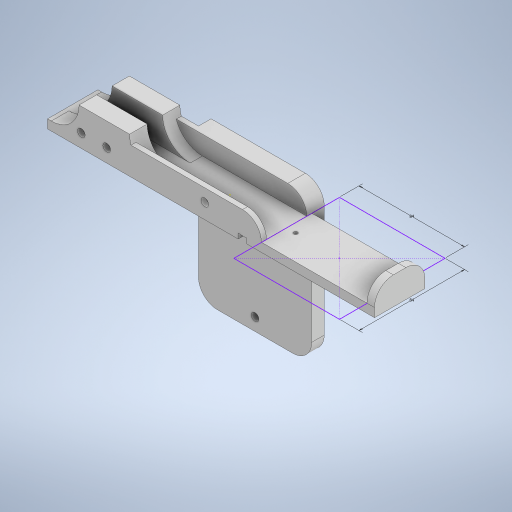
# Autodesk Inventor part: Zeitmessung_Halterung
Saved by Autodesk Inventor 2024.2 (Build 282272000, 272)
## iProperties
Created: 2023-10-20
Part Number: Zeitmessung_Halterung
Material: Generic
Document SubType Name: Modeling
Designer: Rene
Density: 1 g/cm^3
Appearance: Default
Author: Rene
Autodesk Inventor part; units mm, degrees
ref_plane "YZ Plane" through (0, 0, 0) normal (1, 0, 0) x (0, 1, 0)
ref_plane "XZ Plane" through (0, 0, 0) normal (0, 1, 0) x (-1, 0, 0)
ref_plane "XY Plane" through (0, 0, 0) normal (0, 0, 1) x (1, 0, 0)
sketch "Sketch2" plane through (0, 0, 0) normal (0, 1, 0) x (-1, 0, 0)
  line L0 (125, -20) -> (-125, -20)
  line L1 (-125, -20) -> (-125, 20)
  line L2 (-125, 20) -> (125, 20)
  line L3 (125, 20) -> (125, -20)
  line L4 (125, -20) -> (-125, 20) construction
  line L5 (-125, -20) -> (125, 20) construction
  point P0 (0, 0)
  dimension "d0" = 250
  dimension "d1" = 40
  constraints: 12 end point, 2 midpoint, 2 parallel, 1 horizontal, 1 perpendicular
  measures "d0" distance of L1.end L2.end
  measures "d1" distance of L0.end L1.end
extrude "Extrusion1" add sketch "Sketch2" along normal blind 7
sketch "Sketch5" plane through (0, 7, 0) normal (0, 1, 0) x (1, 0, 0)
  line L0 (-100, -6) -> (-59.8, -6)
  line L1 (-59.8, -6) -> (-59.8, 6.25)
  line L2 (-59.8, 6.25) -> (-100, 6.25)
  line L3 (-100, 6.25) -> (-100, -6)
  line L4 (-100, -6) -> (-59.8, 6.25) construction
  line L5 (-59.8, -6) -> (-100, 6.25) construction
  line L6 (-100, 6.5) -> (-100, -6)
  circle A0 centre (-115, 0) radius 3.5 projected
  line L7 (-125, -20) -> (125, -20) projected
  line L8 (-59.8, -6) -> (-100, -6)
  line L9 (-100, -6) -> (-100, -20)
  line L10 (-100, -20) -> (-59.8, -20)
  line L11 (-59.8, -20) -> (-59.8, -6)
  line L12 (125, 20) -> (-125, 20) projected
  line L13 (-59.8, 6.25) -> (-100, 6.25)
  line L14 (-100, 6.25) -> (-100, 20)
  line L15 (-100, 20) -> (-59.8, 20)
  line L16 (-59.8, 20) -> (-59.8, 6.25)
  point P0 (0, 0)
  point P1 (-79.9, 0.125)
  point P2 (-59.8, 20)
  point P3 (-100, 6.25)
  point P4 (-59.8, -20)
  point P5 (-111.5, 0)
  dimension "d18" = 40.2
  dimension "d19" = 12.25
  dimension "d41" = 11.5
  dimension "d42" = 40.2
  constraints: 30 end point, 6 parallel, 3 horizontal, 3 perpendicular, 3 point on line, 2 midpoint, 1 horizontal alignment, 1 other
  measures "d18" distance of L2.end L1.end
  measures "d19" distance of L1.end L0.end
  measures "d41" distance from line of point (-111.5, 0) L14
  measures "d42" distance between parallel lines of L9 L11
extrude "Extrusion4" add sketch "Sketch5" along normal blind 22 contours L0 L11 L7 L9 | L6 L14 L12 L16 L2
sketch "Sketch8" plane through (-125, 0, 20) normal (0, 0, 1) x (1, 0, 0)
  line L0 (65.2, 7) -> (25, 7) projected
  line L1 (25, 7) -> (65.2, 7)
  circle A0 centre (47.0137, 10.6993) radius 1.75
  circle A1 centre (26.8137, 10.7) radius 1.75
  line L2 (48.7637, 10.6999) -> (65.2, 10.6999)
  line L3 (65.2, 7) -> (65.2, 29) projected
  line L4 (26.8, 8.9501) -> (25, 8.9501)
  line L5 (25, 7) -> (25, 29) projected
  point P0 (125, 0)
  dimension "d30" = 3.5
  dimension "d31" = 3.5
  dimension "d32" = 16.7
  dimension "d36" = 3.7
  dimension "d44" = 1.8
  constraints: 6 end point, 3 horizontal, 2 point on line, 6 other
  measures "d36" distance from line of L0 point (26.814, 10.7)
  measures "d44" distance of L4.start L4.end
extrude "Extrusion6" cut sketch "Sketch8" against normal through all
sketch "Sketch9" plane through (0, 7, 0) normal (0, 1, 0) x (1, 0, 0)
  line L0 (61, -11.5) -> (100, -11.5)
  line L1 (100, -11.5) -> (100, 11.5)
  line L2 (100, 11.5) -> (61, 11.5)
  line L3 (61, 11.5) -> (61, -11.5)
  circle A0 centre (80.5, 0) radius 2.05 projected
  line L4 (61, -11.5) -> (100, 11.5) construction
  line L5 (100, -11.5) -> (61, 11.5) construction
  circle A1 centre (115, 0) radius 3.5 projected
  line L6 (-125, -20) -> (125, -20) projected
  line L7 (-59.8, -6) -> (-59.8, -20) projected
  line L8 (125, -20) -> (-59.8, -20)
  line L9 (-59.8, -20) -> (-59.8, -16)
  line L10 (-59.8, -16) -> (125, -16)
  line L11 (125, -16) -> (125, -20)
  line L12 (125, 20) -> (-125, 20) projected
  line L13 (125, 20) -> (-59.8, 20)
  line L14 (-59.8, 20) -> (-59.8, 16)
  line L15 (-59.8, 16) -> (125, 16)
  line L16 (125, 16) -> (125, 20)
  point P0 (0, 0)
  point P1 (-59.8, 20)
  dimension "d39" = 39
  dimension "d40" = 23
  dimension "d45" = 4
  dimension "d46" = 4
  constraints: 28 end point, 6 parallel, 3 horizontal, 3 perpendicular, 2 midpoint, 2 point on line
  measures "d39" distance of L2.end L1.end
  measures "d40" distance of L1.end L0.end
  measures "d45" distance of L8.end L9.end
  measures "d46" distance of L14.end L13.end
extrude "Extrusion7" add sketch "Sketch9" along normal blind 15 contours L7 L10 L11 L6 | L16 L15 L14 L12
fillet "Face Fillet1" radius 22 1 edges at (-100, 7, 13)
fillet "Face Fillet2" radius 21.999 1 edges at (-100, 7, -13.125)
fillet "Face Fillet3" radius 22 1 edges at (-59.8, 7, 11)
fillet "Face Fillet4" radius 21.999 1 edges at (-59.8, 7, -11.125)
sketch "Sketch10" plane through (125, 0, -20) normal (0, 0, -1) x (-1, 0, 0)
  circle A0 centre (202.9863, 10.6993) radius 1.75 projected
  line L0 (204.6029, 13.4993) -> (206.2195, 10.6993)
  line L1 (206.2195, 10.6993) -> (204.6029, 7.8993)
  line L2 (204.6029, 7.8993) -> (201.3697, 7.8993)
  line L3 (201.3697, 7.8993) -> (199.7532, 10.6993)
  line L4 (199.7532, 10.6993) -> (201.3697, 13.4993)
  line L5 (201.3697, 13.4993) -> (204.6029, 13.4993)
  circle A1 centre (223.1863, 10.7) radius 1.75 projected
  line L6 (224.8029, 13.5) -> (226.4195, 10.7)
  line L7 (226.4195, 10.7) -> (224.8029, 7.9)
  line L8 (224.8029, 7.9) -> (221.5697, 7.9)
  line L9 (221.5697, 7.9) -> (219.9532, 10.7)
  line L10 (219.9532, 10.7) -> (221.5697, 13.5)
  line L11 (221.5697, 13.5) -> (224.8029, 13.5)
  point P0 (125, 0)
  dimension "d55" = 5.6
  dimension "d56" = 5.6
  constraints: 24 end point, 2 coincident, 26 other
  measures "d55" distance between parallel lines of L2 L5
  measures "d56" distance between parallel lines of L8 L11
extrude "Extrusion8" cut sketch "Sketch10" against normal blind 5 contours A0 | L0 L1 L2 L3 L4 L5 | A1 | L6 L7 L8 L9 L10 L11
sketch "Sketch11" plane through (-125, 0, 20) normal (0, 0, 1) x (1, 0, 0)
  circle A0 centre (26.8137, 10.7) radius 1.75 projected
  circle A1 centre (26.8137, 10.7) radius 3
  circle A2 centre (47.0137, 10.6993) radius 1.75 projected
  circle A3 centre (47.0137, 10.6993) radius 3
  point P0 (125, 0)
  dimension "d59" = 6
  dimension "d60" = 6
  constraints: 2 centre point, 2 coincident
  measures "d59" diameter of A1
  measures "d60" diameter of A3
extrude "Extrusion9" cut sketch "Sketch11" against normal blind 4
sketch "Sketch24" plane through (125, 0, -20) normal (0, 0, -1) x (-1, 0, 0)
  line L0 (125, 0) -> (170, 0)
  line L1 (0, 0) -> (250, 0) projected
  line L2 (183.6567, 22) -> (0, 22) projected
  line L3 (170, 0) -> (80, 0)
  line L4 (80, 0) -> (80, 22)
  line L5 (80, 22) -> (170, 22)
  line L6 (170, 22) -> (170, 0)
  point P0 (15, 22)
  point P1 (170, 22)
  point P2 (80, 0)
  dimension "d103" = 45
  dimension "d104" = 90
  constraints: 10 end point, 2 parallel, 2 point on line, 1 horizontal, 1 perpendicular
  measures "d103" distance of L0.start L0.end
  measures "d104" distance of L4.end L5.end
extrude "Extrusion20" add sketch "Sketch24" along normal blind 10
sketch "Sketch25" plane through (0, 0, 0) normal (0, -1, 0) x (1, 0, 0)
  line L0 (-45, -30) -> (45, -30) projected
  line L1 (45, -20) -> (45, -30) projected
  line L2 (-45, -30) -> (45, -30)
  line L3 (45, -30) -> (45, -20)
  line L4 (45, -20) -> (-45, -20)
  line L5 (-45, -20) -> (-45, -30)
  point P0 (0, 0)
  constraints: 8 end point, 2 parallel, 1 horizontal, 1 perpendicular
extrude "Extrusion21" add sketch "Sketch25" along normal blind 80
sketch "Sketch28" plane through (125, 0, -30) normal (0, 0, -1) x (-1, 0, 0)
  circle A0 centre (94.9248, -27.5) radius 3.5
  line L0 (170, 22) -> (80, 22) projected
  line L1 (80, 22) -> (80, -80) projected
  point P0 (125, 0)
  point P1 (80, -29)
  dimension "d132" = 7
  dimension "d134" = 46
  dimension "d135" = 15
  constraints: 1 centre point, 1 midpoint
  measures "d132" diameter of A0
  measures "d134" distance edge to line of A0 L0
  measures "d135" distance of A0.centre point (80, -29)
extrude "Extrusion23" cut sketch "Sketch28" against normal up to surface (10 mm away)
sketch "Sketch30" plane through (0, -80, 0) normal (0, -1, 0) x (1, 0, 0)
  line L0 (45, -20) -> (45, -30) projected
  line L1 (45, -20) -> (-45, -20) projected
  line L2 (45, -30) -> (-45, -30)
  line L3 (-45, -30) -> (-45, -20)
  line L4 (-45, -20) -> (45, -20)
  line L5 (45, -20) -> (45, -30)
  point P0 (0, 0)
  constraints: 8 end point, 2 parallel, 1 horizontal, 1 perpendicular
extrude "Extrusion25" add sketch "Sketch30" along normal blind 17
sketch "Sketch31" plane through (125, 0, -30) normal (0, 0, -1) x (-1, 0, 0)
  line L0 (80, -97) -> (170, -97) projected
  line L1 (170, 22) -> (170, -97) projected
  line L2 (80, -97) -> (170, -97)
  line L3 (170, -97) -> (170, -77)
  line L4 (170, -77) -> (80, -77)
  line L5 (80, -77) -> (80, -97)
  circle A0 centre (125, -87) radius 3
  point P0 (125, 0)
  dimension "d143" = 20
  dimension "d144" = 6
  dimension "d170" = 10
  constraints: 8 end point, 2 parallel, 1 centre point, 1 horizontal, 1 perpendicular, 1 point on line
  measures "d143" distance of L3.end L2.end
  measures "d144" diameter of A0
  measures "d170" distance from line of L0 A0.centre
extrude "Extrusion26" cut sketch "Sketch31" against normal through all contours A0
sketch "Sketch35" plane through (-125, 0, 20) normal (0, 0, 1) x (1, 0, 0)
  circle A0 centre (125, 12) radius 3
  line L0 (66.3433, 22) -> (250, 22) projected
  point P0 (125, 0)
  point P1 (125.5, 22)
  point P2 (235, 22)
  dimension "d160" = 6
  dimension "d161" = 10
  constraints: 1 centre point
  measures "d160" diameter of A0
  measures "d161" distance from line of L0 A0.centre
extrude "Extrusion30" cut sketch "Sketch35" against normal blind 4
sketch "Sketch36" plane through (-45, -97, -20) normal (0, 0, 1) x (1, 0, 0)
  circle A0 centre (75.0752, 69.5) radius 3.5 projected
  line L0 (78.5752, 69.5) -> (71.5752, 69.5)
  line L1 (71.5752, 69.5) -> (71.5752, 101)
  line L2 (71.5752, 101) -> (78.5752, 101)
  line L3 (78.5752, 101) -> (78.5752, 69.5)
  point P0 (45, 97)
  point P1 (71.5752, 69.5)
  dimension "d164" = 7
  constraints: 8 end point, 2 parallel, 1 horizontal, 1 perpendicular, 2 other
  measures "d164" distance of L1.end L2.end
extrude "Extrusion31" cut sketch "Sketch36" against normal blind 4 contours A0 L1 L2 L3
sketch "Sketch37" plane through (0, 0, 0) normal (0, -1, 0) x (1, 0, 0)
  line L0 (-58.6567, 20) -> (125, 20) projected
  line L1 (26.5752, -24) -> (33.5752, -24)
  line L2 (33.5752, -24) -> (33.5752, 20)
  line L3 (33.5752, 20) -> (26.5752, 20)
  line L4 (26.5752, 20) -> (26.5752, -24)
  point P0 (0, 0)
  point P1 (0.5, 20)
  point P2 (110, 20)
  dimension "d167" = 7
  constraints: 8 end point, 2 parallel, 1 horizontal, 1 perpendicular, 1 point on line
  measures "d167" distance of L3.end L2.end
extrude "Extrusion32" cut sketch "Sketch37" against normal blind 4
fillet "Rundung5" radius 15 1 edges at (45, -97, -25)
fillet "Rundung6" radius 15 1 edges at (-45, -97, -25)
sketch "Skizze40" plane through (0, 7, 0) normal (0, 1, 0) x (1, 0, 0)
  point P0 (0, 0)
sketch "Skizze41" plane through (0, 7, 0) normal (0, 1, 0) x (1, 0, 0)
  line L0 (125, -20) -> (125, -16) projected
  line L1 (125, -20) -> (135, -20)
  line L2 (135, -20) -> (135, 20)
  line L3 (135, 20) -> (125, 20)
  line L4 (125, 20) -> (125, -20)
  point P0 (0, 0)
  dimension "d173" = 10
  constraints: 8 end point, 2 parallel, 1 horizontal, 1 perpendicular
  measures "d173" distance of L3.end L2.end
extrude "Extrusion33" add sketch "Skizze41" against normal blind 7
sketch "Skizze42" plane through (0, 7, 0) normal (0, 1, 0) x (1, 0, 0)
  line L0 (45, -42) -> (129, -42)
  line L1 (129, -42) -> (129, 42)
  line L2 (129, 42) -> (45, 42)
  line L3 (45, 42) -> (45, -42)
  line L4 (45, -42) -> (129, 42) construction
  line L5 (129, -42) -> (45, 42) construction
  point P0 (0, 0)
  point P1 (87, 0)
  dimension "d176" = 84
  dimension "d177" = 84
  constraints: 12 end point, 2 midpoint, 2 parallel, 1 horizontal, 1 perpendicular
  measures "d176" distance of L2.end L1.end
  measures "d177" distance of L1.end L0.end
sketch "Skizze43" plane through (0, 22, 0) normal (0, 1, 0) x (1, 0, 0)
  line L0 (125, -20) -> (125, -16) projected
  line L1 (-37.8, -16) -> (125, -16) projected
  line L2 (125, -20) -> (45, -20)
  line L3 (45, -20) -> (45, -16)
  line L4 (45, -16) -> (125, -16)
  line L5 (125, -16) -> (125, -20)
  point P0 (0, 0)
  dimension "d178" = 80
  constraints: 8 end point, 2 parallel, 1 horizontal, 1 perpendicular, 1 point on line
  measures "d178" distance of L3.end L4.end
extrude "Extrusion34" cut sketch "Skizze43" against normal blind 15
sketch "Skizze44" plane through (0, 22, 0) normal (0, 1, 0) x (1, 0, 0)
  line L0 (125, 20) -> (45, 20) projected
  line L1 (125, 16) -> (45, 16)
  line L2 (45, 16) -> (45, 20)
  line L3 (45, 20) -> (125, 20)
  line L4 (125, 20) -> (125, 16)
  point P0 (0, 0)
  constraints: 8 end point, 2 parallel, 1 horizontal, 1 perpendicular
extrude "Extrusion35" cut sketch "Skizze44" against normal blind 15
sketch "Skizze45" plane through (0, 7, 0) normal (0, 1, 0) x (1, 0, 0)
  line L0 (135, -20) -> (135, 20) projected
  line L1 (135, -20) -> (45, -20) projected
  line L2 (135, 20) -> (129, 20)
  line L3 (129, 20) -> (129, -20)
  line L4 (129, -20) -> (135, -20)
  line L5 (135, -20) -> (135, 20)
  point P0 (0, 0)
  dimension "d183" = 6
  constraints: 8 end point, 2 parallel, 1 horizontal, 1 perpendicular, 1 point on line
  measures "d183" distance of L4.end L3.end
extrude "Extrusion36" add sketch "Skizze45" along normal blind 15
fillet "Rundung7" radius 15 2 edges at (132, 22, -20) (132, 22, 20)
fillet "Rundung8" radius 15 2 edges at (45, 22, -23) (45, 22, 18)
sketch "Skizze46" plane through (125, 0, -30) normal (0, 0, -1) x (-1, 0, 0)
  circle A0 centre (151, 15) radius 2
  circle A1 centre (151, -70) radius 2
  circle A2 centre (94.9248, -27.5) radius 3.5 projected
  circle A3 centre (105, 15) radius 2
  line L0 (170, 22) -> (95, 22) projected
  circle A4 centre (105, -70) radius 2
  line L1 (80, 7) -> (80, -82) projected
  point P0 (125, 0)
  dimension "d188" = 4
  dimension "d189" = 4
  dimension "d190" = 81
  dimension "d191" = 42.5
  dimension "d192" = 4
  dimension "d193" = 46
  dimension "d194" = 7
  dimension "d195" = 7
  dimension "d196" = 4
  dimension "d197" = 46
  dimension "d198" = 85
  dimension "d214" = 25
  constraints: 4 centre point
  measures "d188" diameter of A0
  measures "d189" diameter of A1
  measures "d191" vertical distance of A2.centre A1.centre
  measures "d192" diameter of A3
  measures "d193" distance of A3.centre A0.centre
  measures "d194" distance from line of L0 A0.centre
  measures "d195" distance from line of L0 A3.centre
  measures "d196" diameter of A4
  measures "d197" distance of A4.centre A1.centre
  measures "d198" distance of A3.centre A4.centre
  measures "d214" distance from line of A4.centre L1
extrude "Extrusion37" cut sketch "Skizze46" against normal blind 7 contours A0 | A1 | A3 | A4
sketch "Skizze47" plane through (0, 7, 0) normal (0, 1, 0) x (1, 0, 0)
  circle A0 centre (121.75, 0) radius 1.5
  line L0 (129, 5) -> (129, -5) projected
  circle A1 centre (52.25, 0) radius 1.5
  line L1 (45, 16) -> (45, 20) projected
  point P0 (0, 0)
  dimension "d201" = 3
  dimension "d202" = 7.25
  dimension "d203" = 3
  dimension "d206" = 69.5
  dimension "d207" = 7.25
  constraints: 2 centre point
  measures "d201" diameter of A0
  measures "d202" distance from line of L0 A0.centre
  measures "d203" diameter of A1
  measures "d206" distance of A0.centre A1.centre
  measures "d207" distance from line of L1 A1.centre
extrude "Extrusion38" cut sketch "Skizze47" against normal blind 10
sketch "Skizze48" plane through (0, 0, 0) normal (0, -1, 0) x (1, 0, 0)
  circle A0 centre (52.25, 0) radius 1.5 projected
  line L0 (49.45, 1.6166) -> (52.25, 3.2332)
  line L1 (52.25, 3.2332) -> (55.05, 1.6166)
  line L2 (55.05, 1.6166) -> (55.05, -1.6166)
  line L3 (55.05, -1.6166) -> (52.25, -3.2332)
  line L4 (52.25, -3.2332) -> (49.45, -1.6166)
  line L5 (49.45, -1.6166) -> (49.45, 1.6166)
  circle A1 centre (121.75, 0) radius 1.5 projected
  line L6 (118.95, 1.6166) -> (121.75, 3.2332)
  line L7 (121.75, 3.2332) -> (124.55, 1.6166)
  line L8 (124.55, 1.6166) -> (124.55, -1.6166)
  line L9 (124.55, -1.6166) -> (121.75, -3.2332)
  line L10 (121.75, -3.2332) -> (118.95, -1.6166)
  line L11 (118.95, -1.6166) -> (118.95, 1.6166)
  point P0 (0, 0)
  dimension "d210" = 5.6
  dimension "d211" = 5.6
  constraints: 24 end point, 2 coincident, 26 other
  measures "d210" distance between parallel lines of L5 L2
  measures "d211" distance between parallel lines of L8 L11
extrude "Extrusion39" cut sketch "Skizze48" against normal blind 2 contours A0 | L0 L1 L2 L3 L4 L5 | A1 | L6 L7 L8 L9 L10 L11
body "Solid1"
